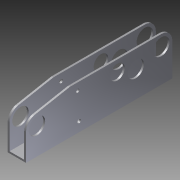
# Autodesk Inventor part: apendage L bracket left
Saved by Autodesk Inventor 2012 (Build 160160000, 160)
## iProperties
Created: 2013-07-07
Part Number: apendage L bracket left
Material: Default
Document SubType Name: Modeling
Designer: Bryce
Density: 1 g/cm^3
Author: Bryce
Autodesk Inventor part; units mm, degrees
ref_plane "YZ Plane" through (0, 0, 0) normal (1, 0, 0) x (0, 1, 0)
ref_plane "XZ Plane" through (0, 0, 0) normal (0, 1, 0) x (-1, 0, 0)
ref_plane "XY Plane" through (0, 0, 0) normal (0, 0, 1) x (1, 0, 0)
sketch "Sketch1" plane through (0, 0, 0) normal (0, 0, 1) x (1, 0, 0)
  line L0 (0, 0) -> (31.75, 0)
  line L1 (0, 76.2) -> (0, 0)
  line L2 (3.175, 3.175) -> (3.175, 76.2)
  line L3 (0, 76.2) -> (3.175, 76.2)
  line L4 (31.75, 76.2) -> (31.75, 0)
  line L5 (31.75, 76.2) -> (28.575, 76.2)
  line L6 (28.575, 76.2) -> (28.575, 3.175)
  line L7 (28.575, 3.175) -> (3.175, 3.175)
  dimension "d0" = 76.2
  dimension "d1" = 31.75
  dimension "d2" = 3.175
  dimension "d20" = 3.175
  dimension "d21" = 3.175
  constraints: 16 end point, 5 perpendicular, 1 horizontal, 1 horizontal alignment, 1 parallel
  measures "d0" distance of L1.start L0.start
  measures "d1" distance of L0.start L0.end
  measures "d2" distance between parallel lines of L1 L2
  measures "d20" distance between parallel lines of L0 L7
  measures "d21" distance between parallel lines of L4 L6
extrude "Extrusion1" add sketch "Sketch1" along normal blind 254
sketch "Sketch2" plane through (3.175, 3.175, 0) normal (1, 0, 0) x (0, 0, -1)
  line L0 (-254, 73.025) -> (-254, 0) projected
  line L1 (0, 73.025) -> (-254, 73.025) projected
  line L2 (0, 73.025) -> (-254, 73.025) projected
  line L3 (0, -3.175) -> (-254, -3.175) projected
  line L4 (-254, 0) -> (-254, -3.175) projected
  line L5 (0, -3.175) -> (0, 0) projected
  circle A0 centre (-164.3834, 60.325) radius 3.175
  line L6 (0, 0) -> (0, 73.025) projected
  arc A1 (0, 53.975) -> (-19.05, 73.025) centre (-19.05, 53.975) ccw
  circle A2 centre (-19.05, 53.975) radius 14.2875
  line L7 (0, 0) -> (-254, 0) projected
  line L8 (-177.8, 73.025) -> (-173.7896, 0) construction
  line L9 (-173.7896, 0) -> (-148.4278, 1.3928) construction
  line L10 (-148.4278, 1.3928) -> (-152.3617, 73.025) construction
  circle A3 centre (-161.8051, 13.3773) radius 3.175
  circle A4 centre (-95.25, 53.975) radius 12.7
  circle A5 centre (-234.95, 42.8625) radius 14.2875
  circle A6 centre (-19.05, 53.975) radius 38.1 construction
  circle A7 centre (-63.5, 42.8625) radius 14.2875
  arc A8 (-238.48, 61.5826) -> (-254, 42.8625) centre (-234.95, 42.8625) ccw
  line L11 (-238.48, 61.5826) -> (-177.8, 73.025)
  dimension "d8" = 76.2
  dimension "d9" = 12.7
  dimension "d13" = 6.35
  dimension "d17" = 19.05
  dimension "d18" = 28.575
  dimension "d22" = 25.4
  dimension "d23" = 12.7
  dimension "d24" = 12.7
  dimension "d25" = 12.7
  dimension "d26" = 6.35
  dimension "d27" = 12.7
  dimension "d28" = 76.2
  dimension "d29" = 25.4
  dimension "d30" = 28.575
  dimension "d31" = 46.0375
  dimension "d32" = 19.05
  dimension "d33" = 76.2
  dimension "d34" = 28.575
  dimension "d35" = 63.5
  constraints: 9 centre point, 8 end point, 6 point on line, 4 coincident, 4 point on circle, 4 tangent, 3 horizontal alignment, 2 perpendicular
  measures "d8" distance from line of L0 L8.start
  measures "d9" distance from line of L1 A0.centre
  measures "d13" diameter of A0
  measures "d17" radius of A1
  measures "d18" diameter of A2
  measures "d22" distance between parallel lines of L10 L8
  measures "d23" distance from line of A0.centre L8
  measures "d24" distance from line of L8 A3.centre
  measures "d25" distance from line of L9 A3.centre
  measures "d26" diameter of A3
  measures "d27" distance from line of point (0, -3.175) L9
  measures "d28" distance of A1.centre A4.centre
  measures "d29" diameter of A4
  measures "d30" diameter of A5
  measures "d31" distance from line of L3 A5.centre
  measures "d32" distance from line of L0 A5.centre
  measures "d33" diameter of A6
  measures "d34" diameter of A7
  measures "d35" distance from line of L6 A7.centre
extrude "Extrusion2" cut sketch "Sketch2" along normal through all both and the other way through all contours L1 L11 A8 L0 | L1 L6 A1 | A0 | A2 | A3 | A4 | A5 | A7
equation "\"d20\" = d2"
equation "\"d21\" = d20"
equation "\"d23\" = 0.5 * d22"
equation "\"d24\" = d23"
equation "\"d26\" = d13"
equation "\"d34\" = d30"
body "Solid1"
